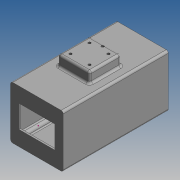
# Autodesk Inventor part: P033_Boitier_v3
Saved by Autodesk Inventor 2021.3 (Build 253353000, 353)
## iProperties
Created: 2021-11-26
Part Number: P033_Boitier_v3
Material: Générique
Document SubType Name: Modeling
Designer: gabri
Density: 1 g/cm^3
Appearance: Par défaut
Author: gabri
Autodesk Inventor part; units mm, degrees
ref_plane "YZ Plane" through (0, 0, 0) normal (1, 0, 0) x (0, 1, 0)
ref_plane "XZ Plane" through (0, 0, 0) normal (0, 1, 0) x (-1, 0, 0)
ref_plane "XY Plane" through (0, 0, 0) normal (0, 0, 1) x (1, 0, 0)
sketch "Sketch3" plane through (0, 0, 0) normal (0, 1, 0) x (-1, 0, 0)
  line L0 (-50, -50) -> (50, -50)
  line L1 (50, -50) -> (50, 50)
  line L2 (50, 50) -> (-50, 50)
  line L3 (-50, 50) -> (-50, -50)
  line L4 (-50, -50) -> (50, 50) construction
  line L5 (50, -50) -> (-50, 50) construction
  point P0 (0, 0)
  dimension "d0" = 100
  dimension "d1" = 100
  constraints: 12 end point, 2 midpoint, 2 parallel, 1 horizontal, 1 perpendicular
  measures "d0" distance between parallel lines of L3 L1
  measures "d1" distance between parallel lines of L0 L2
extrude "Extrusion1" add sketch "Sketch3" along normal blind 200
sketch "Sketch4" plane through (0, 0, 0) normal (0, -1, 0) x (1, 0, 0)
  line L0 (34, -21.5) -> (-34, -21.5)
  line L1 (-34, -21.5) -> (-34, 21.5)
  line L2 (-34, 21.5) -> (34, 21.5)
  line L3 (34, 21.5) -> (34, -21.5)
  line L4 (34, -21.5) -> (-34, 21.5) construction
  line L5 (-34, -21.5) -> (34, 21.5) construction
  point P0 (0, 0)
  dimension "d4" = 68
  dimension "d5" = 43
  constraints: 12 end point, 2 midpoint, 2 parallel, 1 horizontal, 1 perpendicular
  measures "d4" distance of L1.end L2.end
  measures "d5" distance of L0.end L1.end
extrude "Extrusion2" cut sketch "Sketch4" against normal blind 2
shell "Shell1" thickness 3 removed faces 2 at (16.6667, 200, -16.6667) at (-11.3333, 2, -7.1667)
sketch "Sketch10" plane through (0, 200, 0) normal (0, 1, 0) x (1, 0, 0)
  line L0 (-47, 47) -> (-47, -47) construction
  line L1 (-47, -47) -> (47, -47) construction
  line L2 (47, -47) -> (47, 47) construction
  line L3 (47, 47) -> (-47, 47) construction
  line L4 (-50, -50) -> (50, -50) construction
  line L5 (50, -50) -> (50, 50) construction
  line L6 (50, 50) -> (-50, 50) construction
  line L7 (-50, 50) -> (-50, -50) construction
  circle A0 centre (45, -45) radius 5
  circle A1 centre (-45, -45) radius 5
  circle A2 centre (-45, 45) radius 5
  circle A3 centre (45, 45) radius 5
  point P0 (0, 0)
  dimension "d26" = 10
  dimension "d27" = 5
  dimension "d28" = 5
  dimension "d29" = 10
  dimension "d30" = 5
  dimension "d31" = 5
  dimension "d32" = 5
  dimension "d33" = 10
  dimension "d34" = 5
  dimension "d37" = 10
  dimension "d38" = 5
  dimension "d39" = 5
  constraints: 4 centre point
  measures "d26" diameter of A0
  measures "d27" distance from line of L4 A0.centre
  measures "d28" distance from line of A0.centre L5
  measures "d29" diameter of A1
  measures "d30" distance from line of L4 A1.centre
  measures "d31" distance from line of L7 A1.centre
  measures "d32" distance from line of L7 A2.centre
  measures "d33" diameter of A2
  measures "d34" distance from line of L6 A2.centre
  measures "d37" diameter of A3
  measures "d38" distance from line of L5 A3.centre
  measures "d39" distance from line of L6 A3.centre
extrude "Extrusion5" add sketch "Sketch10" against normal up to surface (197 mm away)
sketch "Sketch11" plane through (0, 200, 0) normal (0, 1, 0) x (1, 0, 0)
  line L0 (-40.4174, 47) -> (40.4174, 47) construction
  arc A0 (40.4174, 47) -> (47, 40.4174) centre (45, 45) ccw construction
  line L1 (47, 40.4174) -> (47, -40.4174) construction
  arc A1 (47, -40.4174) -> (40.4174, -47) centre (45, -45) ccw construction
  line L2 (40.4174, -47) -> (-40.4174, -47) construction
  arc A2 (-40.4174, -47) -> (-47, -40.4174) centre (-45, -45) ccw construction
  line L3 (-47, -40.4174) -> (-47, 40.4174) construction
  arc A3 (-47, 40.4174) -> (-40.4174, 47) centre (-45, 45) ccw construction
  line L4 (50, 50) -> (-50, 50) construction
  line L5 (-50, 50) -> (-50, -50) construction
  line L6 (-50, -50) -> (50, -50) construction
  line L7 (50, -50) -> (50, 50) construction
  arc A4 (47, -40.4174) -> (40.4174, -47) centre (45, -45) ccw
  arc A5 (-40.4174, -47) -> (-47, -40.4174) centre (-45, -45) ccw
  arc A6 (-47, 40.4174) -> (-40.4174, 47) centre (-45, 45) ccw
  arc A7 (40.4174, 47) -> (47, 40.4174) centre (45, 45) ccw
  line L8 (40.4174, 47) -> (-40.4174, 47)
  line L9 (47, -40.4174) -> (47, 40.4174)
  line L10 (40.4174, -47) -> (-40.4174, -47)
  line L11 (-47, -40.4174) -> (-47, 40.4174)
  arc A8 (48, -42.3542) -> (42.3542, -48) centre (45, -45) ccw
  line L12 (42.3542, -48) -> (-42.3542, -48)
  arc A9 (-42.3542, -48) -> (-48, -42.3542) centre (-45, -45) ccw
  line L13 (-48, -42.3542) -> (-48, 42.3542)
  arc A10 (-48, 42.3542) -> (-42.3542, 48) centre (-45, 45) ccw
  line L14 (42.3542, 48) -> (-42.3542, 48)
  arc A11 (42.3542, 48) -> (48, 42.3542) centre (45, 45) ccw
  line L15 (48, -42.3542) -> (48, 42.3542)
  point P0 (0, 0)
  dimension "d45" = 1
  dimension "d46" = 4
  dimension "d47" = 1
  dimension "d48" = 4
  dimension "d49" = 1
  dimension "d50" = 4
  dimension "d51" = 1
  dimension "d54" = 4
  constraints: 17 point on circle, 16 end point, 8 centre point, 6 parallel, 4 coincident, 4 concentric, 2 collinear
  measures "d45" distance between parallel lines of L12 L10
  measures "d46" radius of A9
  measures "d47" distance between parallel lines of L13 L3
  measures "d48" radius of A10
  measures "d49" distance between parallel lines of L14 L0
  measures "d50" radius of A11
  measures "d51" distance between parallel lines of L1 L15
  measures "d54" radius of A8
extrude "Extrusion6" add sketch "Sketch11" along normal blind 2
fillet "Fillet1" radius 2 16 edges at (40.4174, 201, 47) (40.4174, 101.5, 47) (47, 201, 40.4174) (47, 101.5, 40.4174) (-40.4174, 201, 47) (-40.4174, 101.5, 47) (-47, 201, 40.4174) (-47, 101.5, 40.4174) (-47, 201, -40.4174) (-47, 101.5, -40.4174) (-40.4174, 201, -47) (-40.4174, 101.5, -47) (40.4174, 201, -47) (40.4174, 101.5, -47) (47, 201, -40.4174) (47, 101.5, -40.4174)
fillet "Fillet2" radius 2 8 edges at (42.3542, 201, -48) (48, 201, -42.3542) (48, 201, 42.3542) (42.3542, 201, 48) (-42.3542, 201, 48) (-48, 201, 42.3542) (-42.3542, 201, -48) (-48, 201, -42.3542)
fillet "Fillet3" radius 0.5 32 edges at (41.4645, 202, 41.4645) (46.4142, 202, 39.4142) (47, 202, 0) (46.4142, 202, -39.4142) (41.4645, 202, -41.4645) (39.4142, 202, -46.4142) (0, 202, -47) (-39.4142, 202, -46.4142) (-41.4645, 202, -41.4645) (-46.4142, 202, -39.4142) (-47, 202, 0) (-46.4142, 202, 39.4142) (-41.4645, 202, 41.4645) (-39.4142, 202, 46.4142) (0, 202, 47) (39.4142, 202, 46.4142) (-40.6114, 202, -47.291) (-42.1716, 202, -42.1716) (-47.291, 202, -40.6114) (-48, 202, 0) (-47.291, 202, 40.6114) (-42.1716, 202, 42.1716) (-40.6114, 202, 47.291) (0, 202, 48) (40.6114, 202, 47.291) (42.1716, 202, 42.1716) (47.291, 202, 40.6114) (48, 202, 0) (47.291, 202, -40.6114) (42.1716, 202, -42.1716) (40.6114, 202, -47.291) (0, 202, -48)
sketch "Sketch12" plane through (0, 200, 0) normal (0, 1, 0) x (1, 0, 0)
  line L0 (-39.0839, 48) -> (39.0839, 48) construction
  arc A0 (41.0559, 45.6667) -> (39.0839, 48) centre (39.0839, 46) ccw construction
  arc A1 (41.0559, 45.6667) -> (45.6667, 41.0559) centre (45, 45) ccw construction
  arc A2 (48, 39.0839) -> (45.6667, 41.0559) centre (46, 39.0839) ccw construction
  line L1 (48, 39.0839) -> (48, -39.0839) construction
  arc A3 (45.6667, -41.0559) -> (48, -39.0839) centre (46, -39.0839) ccw construction
  arc A4 (45.6667, -41.0559) -> (41.0559, -45.6667) centre (45, -45) ccw construction
  arc A5 (39.0839, -48) -> (41.0559, -45.6667) centre (39.0839, -46) ccw construction
  line L2 (39.0839, -48) -> (-39.0839, -48) construction
  arc A6 (-41.0559, -45.6667) -> (-39.0839, -48) centre (-39.0839, -46) ccw construction
  arc A7 (-41.0559, -45.6667) -> (-45.6667, -41.0559) centre (-45, -45) ccw construction
  arc A8 (-48, -39.0839) -> (-45.6667, -41.0559) centre (-46, -39.0839) ccw construction
  line L3 (-48, -39.0839) -> (-48, 39.0839) construction
  arc A9 (-45.6667, 41.0559) -> (-48, 39.0839) centre (-46, 39.0839) ccw construction
  arc A10 (-45.6667, 41.0559) -> (-41.0559, 45.6667) centre (-45, 45) ccw construction
  arc A11 (-39.0839, 48) -> (-41.0559, 45.6667) centre (-39.0839, 46) ccw construction
  line L4 (50, 50) -> (-50, 50) construction
  line L5 (-50, 50) -> (-50, -50) construction
  line L6 (-50, -50) -> (50, -50) construction
  line L7 (50, -50) -> (50, 50) construction
  point P0 (0, 0)
  constraints: 4 coincident
hole "Hole1" at (45, 200, 45) at (-45, 200, 45) at (-45, 200, -45) at (45, 200, -45) direction (0, -1, 0) diameter 4.134 depth 14.2 tip angle 118 thread size "M5x0.8" class "6H" standard "ISO Metric profile"
fillet "Fillet4" radius 4 4 edges at (-50, 100, 50) (50, 100, 50) (50, 100, -50) (-50, 100, -50)
sketch "Sketch15" plane through (-46, 0, 50) normal (0, 0, 1) x (1, 0, 0)
  line L0 (92, 200) -> (92, 0) construction
  line L1 (0, 200) -> (92, 200) construction
  line L2 (0, 0) -> (0, 200) construction
  line L3 (0, 0) -> (92, 0) construction
  line L4 (76, 70) -> (16, 70)
  line L5 (16, 70) -> (16, 130)
  line L6 (16, 130) -> (76, 130)
  line L7 (76, 130) -> (76, 70)
  line L8 (76, 70) -> (16, 130) construction
  line L9 (16, 70) -> (76, 130) construction
  line L10 (46, 242.4) -> (46, -40.4) construction
  point P0 (46, 0)
  point P1 (46, 100)
  point P2 (46, 100)
  dimension "d67" = 60
  dimension "d68" = 60
  dimension "d69" = 200
  dimension "d70" = 100
  constraints: 12 end point, 3 midpoint, 2 parallel, 1 horizontal, 1 perpendicular, 1 point on line
  measures "d67" distance between parallel lines of L7 L5
  measures "d68" distance between parallel lines of L4 L6
  measures "d69" distance between parallel lines of L3 L1
  measures "d70" distance from line of point (46, 100) L1
extrude "Extrusion7" add sketch "Sketch15" along normal blind 20
fillet "Fillet5" radius 4 12 edges at (30, 70, 60) (30, 130, 60) (-30, 130, 60) (-30, 70, 60) (-30, 100, 50) (0, 70, 50) (30, 100, 50) (0, 130, 50) (30, 100, 70) (0, 130, 70) (-30, 100, 70) (0, 70, 70)
sketch "Sketch17" plane through (-38, 3, -47) normal (0, 1, 0) x (1, 0, 0)
  point P0 (38, -47)
sketch "Sketch18" plane through (-38, 3, -47) normal (0, 1, 0) x (1, 0, 0)
  line L0 (1, -22.5) -> (1, -71.5) construction
  line L1 (75, -22.5) -> (1, -22.5) construction
  line L2 (75, -71.5) -> (75, -22.5) construction
  line L3 (1, -71.5) -> (75, -71.5) construction
  arc A0 (85, -9) -> (83, -7) centre (83, -9) ccw construction
  arc A1 (78, -2) -> (83, -7) centre (83, -2) ccw construction
  arc A2 (78, -2) -> (76, 0) centre (76, -2) ccw construction
  line L4 (76, 0) -> (0, 0) construction
  arc A3 (0, 0) -> (-2, -2) centre (0, -2) ccw construction
  arc A4 (-7, -7) -> (-2, -2) centre (-7, -2) ccw construction
  arc A5 (-7, -7) -> (-9, -9) centre (-7, -9) ccw construction
  line L5 (-9, -9) -> (-9, -85) construction
  arc A6 (-9, -85) -> (-7, -87) centre (-7, -85) ccw construction
  arc A7 (-2, -92) -> (-7, -87) centre (-7, -92) ccw construction
  arc A8 (-2, -92) -> (0, -94) centre (0, -92) ccw construction
  line L6 (0, -94) -> (76, -94) construction
  arc A9 (76, -94) -> (78, -92) centre (76, -92) ccw construction
  arc A10 (83, -87) -> (78, -92) centre (83, -92) ccw construction
  arc A11 (83, -87) -> (85, -85) centre (83, -85) ccw construction
  line L7 (85, -85) -> (85, -9) construction
  arc A12 (-2, -92) -> (-7, -87) centre (-7, -92) ccw
  arc A13 (-2, -92) -> (0, -94) centre (0, -92) ccw
  arc A14 (83, -87) -> (78, -92) centre (83, -92) ccw
  arc A15 (76, -94) -> (78, -92) centre (76, -92) ccw
  line L8 (76, -94) -> (0, -94)
  line L9 (-7, -87) -> (83, -87)
  point P0 (38, -47)
  constraints: 11 point on circle, 4 centre point, 4 end point, 3 concentric, 2 tangent, 1 collinear, 1 horizontal
extrude "Extrusion8" add sketch "Sketch18" along normal up to surface (197 mm away)
sketch "Sketch19" plane through (-46, 0, 70) normal (0, 0, 1) x (1, 0, 0)
  line L0 (72, 126) -> (72, 74) construction
  line L1 (20, 126) -> (72, 126) construction
  line L2 (20, 74) -> (20, 126) construction
  line L3 (72, 74) -> (20, 74) construction
  line L4 (46, 242.4) -> (46, -40.4) construction
  line L5 (-24, 0) -> (116, 0) construction
  point P0 (46, 0)
  point P1 (28, 118)
  point P2 (46, 125)
  point P3 (64, 118)
  point P4 (28, 82)
  point P5 (64, 82)
  dimension "d77" = 52
  dimension "d78" = 52
  dimension "d79" = 8
  dimension "d80" = 8
  dimension "d84" = 36
  dimension "d87" = 36
  dimension "d90" = 125
  constraints: 1 horizontal, 1 point on line, 1 vertical, 3 other
  measures "d77" distance between parallel lines of L0 L2
  measures "d78" distance between parallel lines of L3 L1
  measures "d79" distance from line of L1 point (28, 118)
  measures "d80" distance from line of L2 point (28, 118)
  measures "d84" distance of point (28, 118) point (64, 118)
  measures "d87" distance of point (28, 118) point (28, 82)
  measures "d90" distance from line of L5 point (46, 125)
hole "Hole2" at (-18, 118, 70) at (18, 118, 70) at (18, 82, 70) at (-18, 82, 70) at (0, 125, 70) direction (0, 0, -1) diameter 4.917 depth 17.1 tip angle 118 thread size "M6x1" class "6H" standard "ISO Metric profile"
sketch "Sketch20" plane through (-37, 2, 24.5) normal (0, 1, 0) x (1, 0, 0)
  line L0 (3, 46) -> (3, 3) construction
  line L1 (71, 46) -> (3, 46) construction
  line L2 (71, 3) -> (71, 46) construction
  line L3 (3, 3) -> (71, 3) construction
  line L4 (0, 0) -> (74, 0) construction
  line L5 (74, 0) -> (74, 49) construction
  line L6 (74, 49) -> (0, 49) construction
  line L7 (0, 49) -> (0, 0) construction
  line L8 (74, 0) -> (0, 0)
  line L9 (0, 0) -> (0, 49)
  line L10 (0, 49) -> (74, 49)
  line L11 (74, 49) -> (74, 0)
  line L12 (74, 0) -> (0, 49) construction
  line L13 (0, 0) -> (74, 49) construction
  line L14 (71, 3) -> (3, 3)
  line L15 (3, 3) -> (3, 46)
  line L16 (3, 46) -> (71, 46)
  line L17 (71, 46) -> (71, 3)
  line L18 (71, 3) -> (3, 46) construction
  line L19 (3, 3) -> (71, 46) construction
  point P0 (37, 24.5)
  constraints: 24 end point, 4 midpoint, 4 parallel, 2 horizontal, 2 perpendicular
extrude "Extrusion9" add sketch "Sketch20" along normal up to surface (1 mm away)
sketch "Sketch21" plane through (-46, 0, 50) normal (0, 0, 1) x (1, 0, 0)
  line L0 (92, 200) -> (92, 0) construction
  line L1 (0, 200) -> (92, 200) construction
  line L2 (0, 0) -> (0, 200) construction
  line L3 (0, 0) -> (92, 0) construction
  arc A0 (72, 66) -> (80, 74) centre (72, 74) ccw construction
  line L4 (20, 66) -> (72, 66) construction
  arc A1 (12, 74) -> (20, 66) centre (20, 74) ccw construction
  line L5 (12, 126) -> (12, 74) construction
  arc A2 (20, 134) -> (12, 126) centre (20, 126) ccw construction
  line L6 (72, 134) -> (20, 134) construction
  arc A3 (80, 126) -> (72, 134) centre (72, 126) ccw construction
  line L7 (80, 74) -> (80, 126) construction
  line L8 (0, 200) -> (-4, 200) construction
  line L9 (-4, 200) -> (-4, 0) construction
  line L10 (-4, 0) -> (0, 0) construction
  line L11 (0, 0) -> (0, 200) construction
  line L12 (96, 200) -> (92, 200) construction
  line L13 (92, 200) -> (92, 0) construction
  line L14 (92, 0) -> (96, 0) construction
  line L15 (96, 0) -> (96, 200) construction
  line L16 (10, 60) -> (0, 60)
  line L17 (0, 60) -> (0, 30)
  line L18 (0, 30) -> (10, 30)
  line L19 (10, 30) -> (10, 60)
  line L20 (10, 60) -> (0, 30) construction
  line L21 (0, 60) -> (10, 30) construction
  line L22 (92, 60) -> (82, 60)
  line L23 (82, 60) -> (82, 30)
  line L24 (82, 30) -> (92, 30)
  line L25 (92, 30) -> (92, 60)
  line L26 (92, 60) -> (82, 30) construction
  line L27 (82, 60) -> (92, 30) construction
  point P0 (46, 0)
  point P1 (5, 45)
  point P2 (87, 45)
  point P3 (92, 45)
  dimension "d101" = 30
  dimension "d102" = 30
  dimension "d103" = 30
  dimension "d104" = 30
  dimension "d105" = 10
  dimension "d106" = 10
  constraints: 24 end point, 5 midpoint, 4 parallel, 2 horizontal, 2 perpendicular, 2 point on line
  measures "d101" distance between parallel lines of L16 L18
  measures "d102" distance between parallel lines of L22 L24
  measures "d103" distance between parallel lines of L3 L18
  measures "d104" distance between parallel lines of L3 L24
  measures "d105" distance between parallel lines of L0 L23
  measures "d106" distance between parallel lines of L11 L19
extrude "Extrusion10" [suppressed]
fillet "Fillet7" [suppressed]
sketch "Sketch22" plane through (46, 30, 70) normal (1, 0, 0) x (0, 0, -1)
  line L0 (17.0718, 30.1463) -> (17.0718, -0.1463) construction
  arc A0 (16, 30) -> (17.0718, 30.1463) centre (16, 34) ccw construction
  line L1 (16, 30) -> (0, 30) construction
  line L2 (0, 30) -> (0, 0) construction
  line L3 (16, 0) -> (0, 0) construction
  arc A1 (17.0718, -0.1463) -> (16, 0) centre (16, -4) ccw construction
  line L4 (8, 22.5) -> (8, 7.5) construction
  line L5 (11, 22.5) -> (11, 7.5)
  line L6 (5, 7.5) -> (5, 22.5)
  arc A2 (11, 22.5) -> (5, 22.5) centre (8, 22.5) ccw
  arc A3 (5, 7.5) -> (11, 7.5) centre (8, 7.5) ccw
  point P0 (70, -30)
  point P1 (8, 15)
  dimension "d110" = 6
  dimension "d111" = 30
  dimension "d112" = 15
  dimension "d113" = 15
  dimension "d115" = 8
  constraints: 8 end point, 4 point on circle, 4 tangent, 2 centre point, 1 midpoint, 1 parallel, 1 vertical
  measures "d110" distance between parallel lines of L5 L6
  measures "d111" distance of L1.end L2.end
  measures "d112" distance from line of L3 point (8, 15)
  measures "d113" distance of L4.start L4.end
  measures "d115" distance from line of point (8, 15) L2
extrude "Extrusion11" [suppressed]
equation "\"d27\" = 0.5 * d26"
equation "\"d28\" = 0.5 * d26"
equation "\"d30\" = 0.5 * d29"
equation "\"d31\" = 0.5 * d29"
equation "\"d32\" = 0.5 * d33"
equation "\"d34\" = 0.5 * d33"
equation "\"d38\" = 0.5 * d37"
equation "\"d39\" = 0.5 * d37"
equation "\"d70\" = 0.5 * d69"
body "Solid1"
